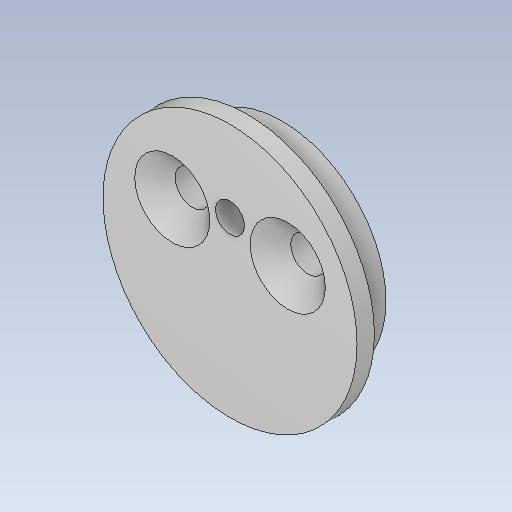
# Autodesk Inventor part: 横回転最終段カム
Saved by Autodesk Inventor 2020 (Build 240168000, 168)
## iProperties
Created: 2019-09-03
Part Number: 横回転最終段カム
Material: アルミニウム 2014-T4
Document SubType Name: Modeling
Designer: tanjihayato
Density: 2.8 g/cm^3
Appearance: サテン
Mass: 3.38187 g
Surface Area: 11.0431 cm^2
Volume: 1.20781 cm^3
Author: tanjihayato
Autodesk Inventor part; units mm, degrees
ref_plane "YZ Plane" through (0, 0, 0) normal (1, 0, 0) x (0, 1, 0)
ref_plane "XZ Plane" through (0, 0, 0) normal (0, 1, 0) x (-1, 0, 0)
ref_plane "XY Plane" through (0, 0, 0) normal (0, 0, 1) x (1, 0, 0)
sketch "スケッチ1" plane through (0, 0, 0) normal (0, 0, 1) x (1, 0, 0)
  circle A0 centre (0, 0) radius 9
  line L0 (-5, 2.8868) -> (5, 2.8868) construction
  line L1 (5, 2.8868) -> (0, -5.7735) construction
  line L2 (0, -5.7735) -> (-5, 2.8868) construction
  circle A1 centre (-5, 2.8868) radius 1.5
  circle A2 centre (5, 2.8868) radius 1.5
  circle A3 centre (0, -5.7735) radius 1.5
  circle A4 centre (0, 4) radius 1.25
  line L3 (0, 0) -> (0, 4) construction
  circle A5 centre (0, 0) radius 10
  dimension "d0" = 18
  dimension "d1" = 10
  dimension "d2" = 3
  dimension "d3" = 3
  dimension "d4" = 3
  dimension "d5" = 2.5
  dimension "d6" = 4
  dimension "d12" = 1
  constraints: 8 end point, 6 centre point, 5 coincident, 1 horizontal, 1 vertical, 7 other
  measures "d0" diameter of A0
  measures "d1" distance of L0.start L0.end
  measures "d2" diameter of A1
  measures "d3" diameter of A2
  measures "d4" diameter of A3
  measures "d5" diameter of A4
  measures "d6" distance of L3.start L3.end
  measures "d12" radial gap between concentric circles of A0 A5
extrude "押し出し1" add sketch "スケッチ1" along normal blind 4.5 contours A0 | A3
sketch "スケッチ2" plane through (0, 0, 4.5) normal (0, 0, 1) x (1, 0, 0)
  circle A0 centre (0, 0) radius 11
  circle A1 centre (5, 2.8868) radius 1.5 projected
  circle A2 centre (-5, 2.8868) radius 1.5 projected
  circle A3 centre (0, 4) radius 1.25 projected
  circle A4 centre (0, 0) radius 9 projected
  dimension "d15" = 2
  constraints: 1 centre point, 1 coincident
  measures "d15" radial gap between concentric circles of A0 A4
extrude "押し出し2" add sketch "スケッチ2" against normal blind 1.5 contours A0
chamfer "面取り2" distance 1.75 angle 45 2 edges at (-6.5, 2.8868, 4.5) (3.5, 2.8868, 4.5)
